Autodesk Fusion 360 part; units mm, degrees
(part 4 of 4)
  arc A226 (29.9244, 6.995) -> (30.8896, 6.995) centre (30.407, 6.995) ccw
  arc A227 (29.9244, 22.235) -> (30.8896, 22.235) centre (30.407, 22.235) ccw
sketch "Sketch2" plane through (0, 0, 0) normal (0, 0, 1) x (1, 0, 0)
  line L0 (11.43, 20.32) -> (7.62, 20.32)
  line L1 (7.62, 11.43) -> (11.43, 11.43)
  line L2 (11.43, 11.43) -> (11.43, 20.32)
  line L3 (7.62, 20.32) -> (7.62, 11.43)
  line L4 (7.62, 24.13) -> (11.43, 24.13)
  line L5 (11.43, 24.13) -> (11.43, 35.56)
  line L6 (7.62, 35.56) -> (7.62, 24.13)
  line L7 (11.43, 35.56) -> (7.62, 35.56)
  line L8 (8.89, 44.45) -> (12.7, 44.45)
  line L9 (8.89, 49.53) -> (8.89, 44.45)
  line L10 (12.7, 44.45) -> (12.7, 49.53)
  line L11 (12.7, 49.53) -> (8.89, 49.53)
  line L12 (23.55, 51.72) -> (23.55, 39.62)
  line L13 (14.55, 39.62) -> (14.55, 51.72)
  line L14 (23.55, 39.62) -> (14.55, 39.62)
  line L15 (14.55, 51.72) -> (23.55, 51.72)
  line L16 (29.21, 17.78) -> (12.7, 17.78)
  line L17 (12.7, 17.78) -> (12.7, 38.1)
  line L18 (29.21, 38.1) -> (29.21, 17.78)
  line L19 (12.7, 38.1) -> (29.21, 38.1)
  line L20 (0, 0) -> (0, 42.188)
  line L21 (35, 0) -> (0, 0)
  line L22 (35, 0) -> (35, 42.1884)
  line L23 (7.62, 20.32) -> (11.43, 11.43) construction
  line L24 (11.43, 20.32) -> (7.62, 11.43) construction
  line L25 (25.5658, 41.294) -> (25.8, 41.0598) construction
  line L26 (25, 44.9968) -> (25.8, 44.6652) construction
  line L27 (25.8, 44.9968) -> (25, 44.6652) construction
  line L28 (27.54, 44.9968) -> (28.3401, 44.6652) construction
  line L29 (28.3401, 44.9968) -> (27.54, 44.6652) construction
  line L30 (27.94, 44.831) -> (25.4, 44.831) construction
  line L31 (25.8, 41.0598) -> (27.54, 40.7282) construction
  line L32 (27.54, 41.0598) -> (25.8, 40.7282) construction
  line L33 (29.205, 17.565) -> (13.205, 17.565)
  line L34 (13.205, 17.565) -> (13.205, 38.665)
  line L35 (13.205, 38.665) -> (29.205, 38.665)
  line L36 (29.205, 38.665) -> (29.205, 17.565)
  line L37 (29.205, 17.565) -> (13.205, 38.665) construction
  line L38 (13.205, 17.565) -> (29.205, 38.665) construction
  line L39 (23.9932, 14.9098) -> (24.2668, 7.9502) construction
  line L40 (23.9932, 7.9502) -> (24.2668, 14.9098) construction
  line L41 (25.38, 7.13) -> (22.88, 7.13)
  line L42 (22.88, 7.13) -> (22.88, 15.73)
  line L43 (22.88, 15.73) -> (25.38, 15.73)
  line L44 (25.38, 15.73) -> (25.38, 7.13)
  line L45 (25.38, 7.13) -> (22.88, 15.73) construction
  line L46 (22.88, 7.13) -> (25.38, 15.73) construction
  line L47 (8.75, 51.7377) -> (26.25, 51.7377)
  line L48 (0, 0) -> (35, 0) construction
  line L49 (35, 0) -> (35, 51.7377) construction
  line L50 (35, 51.7377) -> (0, 51.7377) construction
  line L51 (0, 51.7377) -> (0, 0) construction
  line L52 (-0.3, -0.3) -> (35.3, -0.3)
  line L53 (35.3, -0.3) -> (35.3, 52.0377)
  line L54 (35.3, 52.0377) -> (-0.3, 52.0377)
  line L55 (-0.3, 52.0377) -> (-0.3, -0.3)
  line L56 (10.1791, 41.1868) -> (10.1791, 40.8552)
  line L57 (11.919, 40.8552) -> (11.919, 41.1868)
  line L58 (10.1791, 41.021) -> (11.919, 41.021) construction
  circle A0 centre (26.67, 44.831) radius 2
  line L59 (-1.5, -1.5) -> (36.5, -1.5)
  line L60 (36.5, -1.5) -> (36.5, 53.2377)
  line L61 (36.5, 53.2377) -> (-1.5, 53.2377)
  line L62 (-1.5, 53.2377) -> (-1.5, -1.5)
  circle A1 centre (26.67, 40.894) radius 3.1
  line L63 (7.62, 35.56) -> (11.43, 24.13) construction
  line L64 (7.62, 24.13) -> (11.43, 35.56) construction
  line L65 (12.625, 23.095) -> (6.425, 23.095)
  line L66 (6.425, 23.095) -> (6.425, 36.595)
  line L67 (6.425, 36.595) -> (12.625, 36.595)
  line L68 (12.625, 36.595) -> (12.625, 23.095)
  line L69 (12.625, 23.095) -> (6.425, 36.595) construction
  line L70 (6.425, 23.095) -> (12.625, 36.595) construction
  line L71 (12.625, 10.775) -> (6.425, 10.775)
  line L72 (6.425, 10.775) -> (6.425, 20.975)
  line L73 (6.425, 20.975) -> (12.625, 20.975)
  line L74 (12.625, 20.975) -> (12.625, 10.775)
  line L75 (12.625, 10.775) -> (6.425, 20.975) construction
  line L76 (6.425, 10.775) -> (12.625, 20.975) construction
  line L77 (8.89, 49.53) -> (12.7, 44.45) construction
  line L78 (8.89, 44.45) -> (12.7, 49.53) construction
  line L79 (13.895, 42.99) -> (7.695, 42.99)
  line L80 (7.695, 42.99) -> (7.695, 51.09)
  line L81 (7.695, 51.09) -> (13.895, 51.09)
  line L82 (13.895, 51.09) -> (13.895, 42.99)
  line L83 (13.895, 42.99) -> (7.695, 51.09) construction
  line L84 (7.695, 42.99) -> (13.895, 51.09) construction
  line L85 (14.55, 51.72) -> (23.55, 39.62) construction
  line L86 (14.55, 39.62) -> (23.55, 51.72) construction
  line L87 (23.65, 39.67) -> (14.45, 39.67)
  line L88 (14.45, 39.67) -> (14.45, 51.67)
  line L89 (14.45, 51.67) -> (23.65, 51.67)
  line L90 (23.65, 51.67) -> (23.65, 39.67)
  line L91 (23.65, 39.67) -> (14.45, 51.67) construction
  line L92 (14.45, 39.67) -> (23.65, 51.67) construction
  circle A2 centre (11.049, 41.021) radius 3.2311
  line L93 (11.0268, 42.99) -> (11.0268, 37.79)
  line L94 (13.895, 42.99) -> (13.895, 39.67)
  line L95 (13.895, 39.67) -> (14.45, 39.67)
  line L96 (13.895, 39.67) -> (13.895, 39.4912)
  point P0 (9.525, 15.875)
  point P1 (9.525, 29.845)
  point P2 (10.795, 47.04)
  point P3 (28.1058, 45.2311)
  point P4 (27.7742, 44.431)
  point P5 (27.7742, 45.2311)
  point P6 (27.54, 44.9968)
  point P7 (27.54, 44.6652)
  point P8 (28.1058, 44.431)
  point P9 (28.3401, 44.6652)
  point P10 (28.3401, 44.9968)
  point P11 (25.8, 44.9968)
  point P12 (25.5658, 45.2311)
  point P13 (25.2342, 45.2311)
  point P14 (25, 44.9968)
  point P15 (25, 44.6652)
  point P16 (25.2342, 44.431)
  point P17 (25.5658, 44.431)
  point P18 (25.8, 44.6652)
  point P19 (25.2342, 41.294)
  point P20 (25.5658, 41.294)
  point P21 (25, 41.0598)
  point P22 (25, 40.7282)
  point P23 (25.2342, 40.494)
  point P24 (25.5658, 40.494)
  point P25 (25.8, 40.7282)
  point P26 (25.8, 41.0598)
  point P27 (27.54, 41.0598)
  point P28 (28.1058, 41.294)
  point P29 (27.7742, 41.294)
  point P30 (27.7742, 40.494)
  point P31 (27.54, 40.7282)
  point P32 (28.1058, 40.494)
  point P33 (28.3401, 40.7282)
  point P34 (28.3401, 41.0598)
  point P35 (23.7998, 15.3768)
  point P36 (23.9932, 15.5702)
  point P37 (24.2668, 15.5702)
  point P38 (24.4602, 15.3768)
  point P39 (24.4602, 15.1032)
  point P40 (24.2668, 14.9098)
  point P41 (23.9932, 14.9098)
  point P42 (23.7998, 15.1032)
  point P43 (24.2668, 7.9502)
  point P44 (23.9932, 7.9502)
  point P45 (23.7998, 7.7568)
  point P46 (23.7998, 7.4832)
  point P47 (23.9932, 7.2898)
  point P48 (24.2668, 7.2898)
  point P49 (24.4602, 7.4832)
  point P50 (24.4602, 7.7568)
  point P51 (25.4, 44.831)
  point P52 (21.205, 28.115)
  point P53 (24.13, 11.43)
  point P54 (9.525, 29.845)
  point P55 (9.525, 15.875)
  point P56 (10.795, 47.04)
  point P57 (19.05, 45.67)
  dimension "d9" = 16
  dimension "d10" = 21.1
  dimension "d11" = 2.5
  dimension "d12" = 8.6
  dimension "d13" = 0.3
  dimension "d14" = 4
  dimension "d33" = 1.5
  dimension "d40" = 6.2
  dimension "d41" = 6.2
  dimension "d42" = 13.5
  dimension "d43" = 6.2
  dimension "d44" = 10.2
  dimension "d45" = 6.2
  dimension "d46" = 8.1
  dimension "d47" = 9.2
  dimension "d48" = 12
  dimension "d57" = 5.2
  constraint coincident L0.end L3.start
  constraint coincident L1.end L2.start
  constraint coincident L0.start L2.end
  constraint coincident L1.start L3.end
  constraint midpoint L23 P55
  constraint coincident P14 L26.start
  constraint coincident P18 L26.end
  constraint coincident P11 L27.start
  constraint coincident P15 L27.end
  constraint midpoint L26 P51
  constraint coincident P6 L28.start
  constraint coincident P9 L28.end
  constraint coincident P10 L29.start
  constraint coincident P7 L29.end
  constraint midpoint L29 L30.start
  constraint coincident P51 L30.end
  constraint coincident P26 L25.end
  constraint coincident P31 L31.end
  constraint coincident P27 L32.start
  constraint coincident P25 L32.end
  constraint horizontal L33
  constraint perpendicular L33 L34
  constraint parallel L33 L35
  constraint parallel L34 L36
  constraint coincident L37 P52
  constraint coincident L38 P52
  constraint coincident P41 L39.start
  constraint coincident P43 L39.end
  constraint coincident P44 L40.start
  constraint coincident P40 L40.end
  constraint horizontal L41
  constraint perpendicular L41 L42
  constraint parallel L41 L43
  constraint parallel L42 L44
  constraint coincident L45 P53
  constraint coincident L46 P53
  constraint midpoint L39 P53
  constraint horizontal L48
  constraint vertical L49
  constraint horizontal L50
  constraint vertical L51
  constraint coincident L20.start L21.end
  constraint midpoint L56 L58.start
  constraint midpoint L57 L58.end
  constraint midpoint L30 A0.centre
  constraint midpoint L32 A1.centre
  constraint coincident L6.start L7.end
  constraint coincident L4.end L5.start
  constraint coincident L4.start L6.end
  constraint coincident L5.end L7.start
  constraint horizontal L65
  constraint perpendicular L65 L66
  constraint parallel L65 L67
  constraint parallel L66 L68
  constraint coincident L69 P54
  constraint coincident L70 P54
  constraint coincident P54 P1
  constraint horizontal L71
  constraint perpendicular L71 L72
  constraint parallel L71 L73
  constraint parallel L72 L74
  constraint coincident L75 P55
  constraint coincident L76 P55
  constraint coincident P55 P0
  constraint coincident L9.start L11.end
  constraint coincident L8.end L10.start
  constraint coincident L8.start L9.end
  constraint coincident L10.end L11.start
  constraint horizontal L79
  constraint perpendicular L79 L80
  constraint parallel L79 L81
  constraint parallel L80 L82
  constraint coincident L83 P56
  constraint coincident L84 P56
  constraint coincident P56 P2
  constraint coincident L13.end L15.start
  constraint coincident L12.end L14.start
  constraint coincident L13.start L14.end
  constraint coincident L12.start L15.end
  constraint horizontal L87
  constraint perpendicular L87 L88
  constraint parallel L87 L89
  constraint parallel L88 L90
  constraint coincident L91 P57
  constraint coincident L92 P57
  constraint midpoint L85 P57
  constraint midpoint L58 A2.centre
  constraint coincident L79 L93.start
  constraint coincident A2 L93.end
  constraint perpendicular L58 L93
  constraint perpendicular L87 L94
  constraint perpendicular L13 L95
  constraint coincident A2 L96.end
  constraint perpendicular L95 L96
  measures "d9" distance of L34.end L35.end
  measures "d10" distance of L33.end L34.end
  measures "d11" distance of L42.end L43.end
  measures "d12" distance of L41.end L42.end
  measures "d14" diameter of A0
  measures "d40" diameter of A1
  measures "d41" distance of L66.end L67.end
  measures "d42" distance of L65.end L66.end
  measures "d43" distance of L72.end L73.end
  measures "d44" distance of L71.end L72.end
  measures "d45" distance of L80.end L81.end
  measures "d46" distance of L79.end L80.end
  measures "d47" distance of L88.end L89.end
  measures "d48" distance of L87.end L88.end
  measures "d57" distance of L93.start L93.end
extrude "Extrude1" add sketch "Sketch2" against normal blind 14 contours L0 L1 L2 L3 | L4 L5 L6 L7 | L8 L9 L10 L11 | L12 L13 L15 L89 | L12 A1 L87 L89 L90 | L12 L13 L87 L89 | L12 L13 L14 L35 A1 L87 L90 A2 L95 | L12 L13 L14 L87 | L13 L87 L88 L89 | A1 L90 | L35 A0 A1 L90 | A0 A1 | A0 A1 | L19 L34 L35 A1 A2 | L19 L35 A1 | A2 L94 L95 | A2 L95 L96 | L34 L35 A2 | L34 L35 L79 A2 L93 L94 L96 | L19 L35 L36 A1 | L16 L19 L34 L36 A1 | L19 A1 | L16 L17 L19 L34 | L79 A2 L94 | L79 A2 L93 | L16 L18 L19 L36 | L16 L33 L34 L36 | L79 L80 L81 L82 A2 | L79 A2 | L41 L42 L43 L44 | L52 L53 L54 L55 | L65 L66 L67 L68 | L71 L72 L73 L74
extrude "Extrude2" cut sketch "Sketch2" against normal blind 7 contours L0 L1 L2 L3 | L4 L5 L6 L7 | L8 L9 L10 L11 | L79 L80 L81 L82 A2 | L79 A2 | L65 L66 L67 L68 | L71 L72 L73 L74
extrude "Extrude3" cut sketch "Sketch2" against normal blind 10.4 contours L12 L13 L87 L89
extrude "Extrude4" cut sketch "Sketch2" against normal blind 3 contours A0 A1 | A0 A1
extrude "Extrude5" cut sketch "Sketch2" against normal blind 3 contours L41 L42 L43 L44
extrude "Extrude6" cut sketch "Sketch2" against normal blind 6 contours L19 L34 L35 A1 A2 | L19 L35 A1 | L34 L35 A2 | L19 L35 L36 A1 | L16 L19 L34 L36 A1 | L19 A1 | L16 L33 L34 L36
sketch "Sketch4" plane through (0, 0, -6) normal (0, 0, 1) x (-1, 0, 0)
  line L0 (-13.205, -38.665) -> (-13.205, -17.565)
  line L1 (-29.205, -17.565) -> (-29.205, -38.665)
  line L2 (-13.205, -38.665) -> (-15.705, -38.665)
  line L3 (-13.205, -21.665) -> (-13.205, -38.665)
  line L4 (-13.205, -38.665) -> (-20.705, -38.665)
  line L5 (-13.205, -36.165) -> (-13.205, -38.665)
  line L6 (-13.205, -17.565) -> (-29.205, -17.565)
  line L7 (-29.205, -38.665) -> (-13.205, -38.665)
  line L8 (-29.205, -38.665) -> (-21.705, -38.665)
  line L9 (-21.705, -38.665) -> (-21.705, -35.665)
  line L10 (-21.705, -35.665) -> (-29.205, -35.665)
  line L11 (-29.205, -35.665) -> (-29.205, -38.665)
  line L12 (-29.205, -38.665) -> (-26.205, -38.665)
  line L13 (-26.205, -38.665) -> (-26.205, -21.665)
  line L14 (-26.205, -21.665) -> (-29.205, -21.665)
  line L15 (-29.205, -21.665) -> (-29.205, -38.665)
  dimension "d49" = 7.5
  dimension "d50" = 3
  dimension "d51" = 3
  dimension "d52" = 17
  constraint horizontal L2
  constraint vertical L3
  constraint coincident L0.start L2.start
  constraint horizontal L4
  constraint vertical L5
  constraint horizontal L8
  constraint vertical L9
  constraint horizontal L10
  constraint vertical L11
  constraint coincident L1.end L7.start
  constraint horizontal L12
  constraint vertical L13
  constraint horizontal L14
  constraint vertical L15
  measures "d49" distance of L1.end L8.end
  measures "d50" distance of L1.end L10.end
  measures "d51" distance of L1.end L12.end
  measures "d52" distance of L1.end L14.end
extrude "Extrude7" cut sketch "Sketch4" against normal blind 5.5 contours L7 L8 L9 L10 L13 | L1 L7 L8 L10 L11 L12 L13 L15 | L1 L10 L13 L14 L15
extrude "Extrude9" add sketch "Sketch2" against normal blind 14 contours L59 L60 L61 L62
extrude "Extrude10" cut 1 faces at (13.895, 48.39, -2.3333) along direction (1, 0, 0) blind 1
move_face "OffsetFaces1" offset -0.1 3 faces at (20.55, 39.67, -3.4667) (23.55, 47.67, -3.4667) (20.55, 51.67, -6.9333)
extrude "Extrude11" cut sketch "Sketch2" against normal blind 13 contours A1 L90 | L35 A0 A1 L90 | A0 A1 picked at (26.9042, 43.6048)
extrude "Extrude12" cut sketch "Sketch2" against normal blind 13 contours L34 L35 L79 A2 L93 L94 L96 | L79 A2 L93 | L79 A2
sketch "Sketch5" plane through (0, 0, 0) normal (1, 0, 0) x (0, 1, 0)
fillet "Fillet2" radius 2 4 edges at (36.5, -1.5, -7) (36.5, 53.2377, -7) (-1.5, 53.2377, -7) (-1.5, -1.5, -7)
move_face "OffsetFaces3" offset 0.4 1 faces at (7.695, 45.69, -2.3333)
equation "d33 = ( 0.6 * 2 ) * 1 mm + 0.3 mm"
